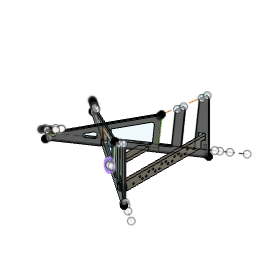
laptop-stand (Autodesk Fusion 360 design; units mm, degrees)
Autodesk Fusion 360 part; units mm, degrees
(part 1 of 2)
sketch "Side-Master" plane through (0, 0, 0) normal (0, 1, 0) x (1, 0, 0) in component "MainPanelRight"
  line L0 (8.1062, 0) -> (397.2, 0)
  line L1 (15.0761, -30.319) -> (18.2492, -20.8358)
  line L2 (13.8069, -34.1123) -> (25, -34.1123) construction
  line L3 (277.5681, -20) -> (310.5681, -20)
  line L4 (277.5681, -20) -> (284.9108, -103.9275)
  line L5 (277.5681, -20) -> (278, -20) construction
  line L6 (277.5681, -20) -> (277.5681, 0) construction
  line L7 (18.2492, -20.8358) -> (279.6598, -108.0704)
  line L8 (310.5681, -20) -> (428, -20) construction
  line L9 (332.9681, -20) -> (365.9681, -20)
  line L10 (365.9681, -20) -> (379.1493, -170.6626)
  line L11 (365.9681, -20) -> (495.2, -20) construction
  line L12 (381.4538, -174.4501) -> (395.0588, -183.0721) construction
  line L13 (401.2, -4) -> (401.2, -179.6934)
  line L14 (-0.6166, -29.9937) -> (35.0053, -29.9937) construction
  line L15 (13.8069, -34.1123) -> (37.7388, -34.1123) construction
  line L16 (13.8069, -34.1123) -> (-9.9012, -26.1797) construction
  line L17 (13.8069, -34.1123) -> (40, -34.1123) construction
  line L18 (0.3599, -26.0548) -> (4.1611, -3.3398)
  line L19 (-0.204, -29.4243) -> (25.3133, -29.4243) construction
  line L20 (3.0358, -30.5083) -> (10.0136, -32.8431)
  line L21 (0, 0) -> (138.5, 0) construction
  line L22 (138.5, 0) -> (138.5, -20.0011) construction
  line L23 (0, -20) -> (0, 0) construction
  line L24 (138.5, -20.0011) -> (138.4351, -60.9427) construction
  line L25 (147.5, -20.0011) -> (147.4778, -63.9603) construction
  line L26 (147.5, -20.0011) -> (147.5, 0) construction
  arc A0 (279.6598, -108.0704) -> (284.9108, -103.9275) centre (280.926, -104.2761) ccw
  arc A1 (379.1493, -170.6626) -> (381.4538, -174.4501) centre (384.1303, -170.2268) ccw
  arc A2 (395.0588, -183.0721) -> (401.2, -179.6934) centre (397.2, -179.6934) ccw
  arc A3 (401.2, -4) -> (397.2, 0) centre (397.2, -4) ccw
  arc A4 (0.3599, -26.0548) -> (3.0358, -30.5083) centre (4.305, -26.715) ccw
  arc A5 (8.1062, 0) -> (4.1611, -3.3398) centre (8.1062, -4) ccw
  arc A6 (10.0136, -32.8431) -> (15.0761, -30.319) centre (11.2828, -29.0498) ccw
  line L27 (285.442, -110) -> (379.1965, -169.4156) construction
  line L28 (310.5681, -20) -> (320.2067, -130.1699)
  line L29 (310.5681, -20) -> (415.8497, -20) construction
  line L30 (332.9681, -20) -> (343.3891, -139.1136)
  line L31 (332.9681, -20) -> (452.9694, -20) construction
  line L32 (322.0503, -133.1999) -> (337.2632, -142.8409)
  arc A7 (320.2067, -130.1699) -> (322.0503, -133.1999) centre (324.1914, -129.8213) ccw
  arc A8 (337.2632, -142.8409) -> (343.3891, -139.1136) centre (339.4044, -139.4622) ccw
  line L33 (381.4538, -174.4501) -> (395.0588, -183.0721)
  line L34 (278, -20) -> (0, -20) construction
  line L35 (310.5681, -20) -> (332.9681, -20) construction
  line L36 (277.5681, -20) -> (257.5681, -20) construction
  line L37 (257.5681, -20) -> (257.5681, -10) construction
  line L38 (257.5681, -10) -> (277.5681, -10) construction
  line L39 (277.5681, -10) -> (277.5681, -20) construction
  line L40 (395.2, -20) -> (390.2, -20) construction
  line L41 (390.2, -20) -> (390.2, -35) construction
  line L42 (390.2, -35) -> (395.2, -35) construction
  line L43 (395.2, -35) -> (395.2, -20) construction
  point P0 (401.2, 0)
  point P1 (285.442, -110)
  dimension "d1" = 401.2
  dimension "d5" = 30
  dimension "d8_1" = 15
  dimension "d9_1" = 71.5
  dimension "d10_1" = 14
  dimension "d11_1" = 33
  dimension "d12_1" = 85
  dimension "d14" = 20
  dimension "d15" = 90
  dimension "d24" = 33
  dimension "d25" = 85
  dimension "d26" = 150
  dimension "d41" = 161.5
  dimension "d42" = 25
  dimension "d44" = 80.5
  dimension "d66" = 138.5
  dimension "d67" = 20
  dimension "d68" = 9
  dimension "d129" = 4
  dimension "d130" = 5
  dimension "d131" = 4
  dimension "d134" = 4
  dimension "d137" = 4
  dimension "d138" = 4
  dimension "d139" = 4
  dimension "d140" = 85
  dimension "d141" = 85
  dimension "d142" = 4
  dimension "d143" = 4
  dimension "d146" = 22.4
  dimension "d38" = 20
  dimension "d39" = 10
  dimension "d53" = 5
  dimension "d54" = 15
  dimension "d156" = 6
  constraint horizontal L0
  constraint coincident L21.start L23.end
  constraint horizontal L2
  constraint horizontal L3
  constraint horizontal L5
  constraint coincident L0 L6.end
  constraint perpendicular L0 L6
  constraint horizontal L8
  constraint parallel L8 L9
  constraint horizontal L11
  constraint horizontal L14
  constraint horizontal L15
  constraint horizontal L17
  constraint horizontal L19
  constraint coincident L16 L19.start
  constraint horizontal L21
  constraint vertical L22
  constraint vertical L23
  constraint coincident L7 L24.end
  constraint coincident L7 L25.end
  constraint coincident L0 L26.end
  constraint perpendicular L0 L26
  constraint coincident P1 L7
  constraint coincident P1 L4
  constraint tangent L7 A0
  constraint tangent L4 A0
  constraint tangent L10 A1
  constraint tangent L12 A1
  constraint tangent L12 A2
  constraint tangent L13 A2
  constraint coincident P0 L13
  constraint coincident P0 L0
  constraint tangent L13 A3
  constraint tangent L0 A3
  constraint coincident L19.start L20
  constraint coincident L19.start L18
  constraint tangent L20 A4
  constraint tangent L18 A4
  constraint coincident L21.start L0
  constraint tangent L18 A5
  constraint tangent L0 A5
  constraint coincident L2.start L20
  constraint coincident L2.start L1
  constraint tangent L20 A6
  constraint tangent L1 A6
  constraint coincident P1 L27.start
  constraint horizontal L29
  constraint horizontal L31
  constraint tangent L28 A7
  constraint tangent L32 A7
  constraint tangent L32 A8
  constraint tangent L30 A8
  constraint perpendicular L23 L34
  constraint parallel L29 L35
  constraint collinear L27 L32
  constraint coincident L27.end A1
  constraint parallel L27 L33
  constraint horizontal L36
  constraint vertical L37
  constraint horizontal L38
  constraint vertical L39
  constraint horizontal L40
  constraint vertical L41
  constraint horizontal L42
  constraint vertical L43
  constraint coincident L31 L40.start
  constraint vertical L13
  measures "d1" distance of L21.start P0
  measures "d5" distance of L21.start L14.start
  measures "d8_1" distance of L14.start L2.start
  measures "d9_1" angle of L1 L2
  measures "d10_1" distance of L2.start L1.end
  measures "d11_1" distance of L3.start L3.end
  measures "d12_1" angle of L4 L5
  measures "d14" distance of L0 L3
  measures "d15" vertical distance of L3.start P1
  measures "d24" distance of L9.start L9.end
  measures "d25" angle of L10 L11
  measures "d26" distance of L9.end L27.end
  measures "d41" angle of L16 L17
  measures "d42" distance of L2.start L16.end
  measures "d44" angle of L18 L19
  measures "d66" distance of L21.start L21.end
  measures "d67" distance of L21.start L23.start
  measures "d68" distance of L22.end L25.start
  measures "d129" radius of A0
  measures "d130" radius of A1
  measures "d131" radius of A2
  measures "d134" radius of A3
  measures "d137" radius of A4
  measures "d138" radius of A5
  measures "d139" radius of A6
  measures "d140" angle of L28 L29
  measures "d141" angle of L30 L31
  measures "d142" radius of A7
  measures "d143" radius of A8
  measures "d146" distance of L3.end L9.start
  measures "d38" distance of L3.start L36.end
  measures "d39" distance of L3.start L38.end
  measures "d53" distance of L40.start L40.end
  measures "d54" distance of L40.start L42.end
  measures "d156" distance of L13 L43
extrude "Extrude24" add sketch "Side-Master" along normal mid plane 9 makes body 1 in component "MainPanelRight"
sketch "Sketch12" plane through (0, 0, 0) normal (0, 0, -1) x (1, 0, 0) in component "MainPanelRight"
  line L0 (8.1062, 4.5) -> (8.1062, -4.5)
  line L1 (8.1062, -4.5) -> (397.2, -4.5)
  line L2 (397.2, -4.5) -> (397.2, 4.5)
  line L3 (397.2, 4.5) -> (8.1062, 4.5)
  line L4 (397.2, 0) -> (401.2, 0) construction
  dimension "d149" = 4
  constraint midpoint L2 L4.start
  constraint perpendicular L2 L4
  measures "d149" distance of L4.start L4.end
sketch "Side-Master (2)" plane through (0, 0, 0) normal (0, 1, 0) x (1, 0, 0) in component "MainPanelLeft"
  line L0 (8.1062, 0) -> (397.2, 0)
  line L1 (15.0761, -30.319) -> (18.2492, -20.8358)
  line L2 (13.8069, -34.1123) -> (25, -34.1123) construction
  line L3 (277.5681, -20) -> (310.5681, -20)
  line L4 (277.5681, -20) -> (284.9108, -103.9275)
  line L5 (277.5681, -20) -> (278, -20) construction
  line L6 (277.5681, -20) -> (277.5681, 0) construction
  line L7 (18.2492, -20.8358) -> (279.6598, -108.0704)
  line L8 (310.5681, -20) -> (428, -20) construction
  line L9 (332.9681, -20) -> (365.9681, -20)
  line L10 (365.9681, -20) -> (379.1479, -170.6469)
  line L11 (365.9681, -20) -> (495.2, -20) construction
  line L12 (381.4524, -174.4344) -> (395.0587, -183.0577) construction
  line L13 (401.2, -4) -> (401.2, -179.6791)
  line L14 (-0.6166, -29.9937) -> (35.0053, -29.9937) construction
  line L15 (13.8069, -34.1123) -> (37.7388, -34.1123) construction
  line L16 (13.8069, -34.1123) -> (-9.9012, -26.1797) construction
  line L17 (13.8069, -34.1123) -> (40, -34.1123) construction
  line L18 (0.3599, -26.0548) -> (4.1611, -3.3398)
  line L19 (-0.204, -29.4243) -> (25.3133, -29.4243) construction
  line L20 (3.0358, -30.5083) -> (10.0136, -32.8431)
  line L21 (0, 0) -> (138.5, 0) construction
  line L22 (138.5, 0) -> (138.5, -20.0011) construction
  line L23 (0, -20) -> (0, 0) construction
  line L24 (138.5, -20.0011) -> (138.4351, -60.9427) construction
  line L25 (147.5, -20.0011) -> (147.4778, -63.9603) construction
  line L26 (147.5, -20.0011) -> (147.5, 0) construction
  arc A0 (279.6598, -108.0704) -> (284.9108, -103.9275) centre (280.926, -104.2761) ccw
  arc A1 (379.1479, -170.6469) -> (381.4524, -174.4344) centre (384.1289, -170.2111) ccw
  arc A2 (395.0587, -183.0577) -> (401.2, -179.6791) centre (397.2, -179.6791) ccw
  arc A3 (401.2, -4) -> (397.2, 0) centre (397.2, -4) ccw
  arc A4 (0.3599, -26.0548) -> (3.0358, -30.5083) centre (4.305, -26.715) ccw
  arc A5 (8.1062, 0) -> (4.1611, -3.3398) centre (8.1062, -4) ccw
  arc A6 (10.0136, -32.8431) -> (15.0761, -30.319) centre (11.2828, -29.0498) ccw
  line L27 (285.442, -110) -> (379.1926, -169.4159) construction
  line L28 (310.5681, -20) -> (320.2068, -130.1711)
  line L29 (310.5681, -20) -> (415.8497, -20) construction
  line L30 (332.9681, -20) -> (343.3893, -139.1153)
  line L31 (332.9681, -20) -> (452.9694, -20) construction
  line L32 (322.0503, -133.2011) -> (337.2633, -142.8425)
  arc A7 (320.2068, -130.1711) -> (322.0503, -133.2011) centre (324.1916, -129.8225) ccw
  arc A8 (337.2633, -142.8425) -> (343.3893, -139.1153) centre (339.4045, -139.4639) ccw
  line L33 (381.4524, -174.4344) -> (395.0587, -183.0577)
  line L34 (278, -20) -> (0, -20) construction
  line L35 (310.5681, -20) -> (332.9681, -20) construction
  line L36 (277.5681, -20) -> (257.5681, -20) construction
  line L37 (257.5681, -20) -> (257.5681, -10) construction
  line L38 (257.5681, -10) -> (277.5681, -10) construction
  line L39 (277.5681, -10) -> (277.5681, -20) construction
  line L40 (257.5681, -10) -> (247.5681, -10) construction
  line L41 (395.2, -20) -> (390.2, -20) construction
  line L42 (390.2, -20) -> (390.2, -35) construction
  line L43 (390.2, -35) -> (395.2, -35) construction
  line L44 (395.2, -35) -> (395.2, -20) construction
  line L45 (390.2, -35) -> (390.2, -45) construction
  point P0 (401.2, 0)
  point P1 (285.442, -110)
  dimension "d1_1" = 401.2
  dimension "d5_1" = 30
  dimension "d8_2" = 15
  dimension "d9_2" = 71.5
  dimension "d10_2" = 14
  dimension "d11_2" = 33
  dimension "d12_2" = 85
  dimension "d14_1" = 20
  dimension "d15_1" = 90
  dimension "d24_1" = 33
  dimension "d25_1" = 85
  dimension "d26_1" = 150
  dimension "d41_1" = 161.5
  dimension "d42_1" = 25
  dimension "d44_1" = 80.5
  dimension "d66_1" = 138.5
  dimension "d67_1" = 20
  dimension "d68_1" = 9
  dimension "d129_1" = 4
  dimension "d130_1" = 5
  dimension "d131_1" = 4
  dimension "d134_1" = 4
  dimension "d137_1" = 4
  dimension "d138_1" = 4
  dimension "d139_1" = 4
  dimension "d140_1" = 85
  dimension "d141_1" = 85
  dimension "d142_1" = 4
  dimension "d143_1" = 4
  dimension "d146_1" = 22.4
  dimension "d37" = 20
  dimension "d40" = 10
  dimension "d50" = 5
  dimension "d51" = 15
  dimension "d52" = 10
  dimension "d155" = 6
  constraint horizontal L0
  constraint coincident L21.start L23.end
  constraint horizontal L2
  constraint horizontal L3
  constraint horizontal L5
  constraint coincident L0 L6.end
  constraint perpendicular L0 L6
  constraint horizontal L8
  constraint parallel L8 L9
  constraint horizontal L11
  constraint horizontal L14
  constraint horizontal L15
  constraint horizontal L17
  constraint horizontal L19
  constraint coincident L16 L19.start
  constraint horizontal L21
  constraint vertical L22
  constraint vertical L23
  constraint coincident L7 L24.end
  constraint coincident L7 L25.end
  constraint coincident L0 L26.end
  constraint perpendicular L0 L26
  constraint coincident P1 L7
  constraint coincident P1 L4
  constraint tangent L7 A0
  constraint tangent L4 A0
  constraint tangent L10 A1
  constraint tangent L12 A1
  constraint tangent L12 A2
  constraint tangent L13 A2
  constraint coincident P0 L13
  constraint coincident P0 L0
  constraint tangent L13 A3
  constraint tangent L0 A3
  constraint coincident L19.start L20
  constraint coincident L19.start L18
  constraint tangent L20 A4
  constraint tangent L18 A4
  constraint coincident L21.start L0
  constraint tangent L18 A5
  constraint tangent L0 A5
  constraint coincident L2.start L20
  constraint coincident L2.start L1
  constraint tangent L20 A6
  constraint tangent L1 A6
  constraint coincident P1 L27.start
  constraint horizontal L29
  constraint horizontal L31
  constraint tangent L28 A7
  constraint tangent L32 A7
  constraint tangent L32 A8
  constraint tangent L30 A8
  constraint perpendicular L23 L34
  constraint parallel L29 L35
  constraint collinear L27 L32
  constraint coincident L27.end A1
  constraint parallel L27 L33
  constraint horizontal L36
  constraint vertical L37
  constraint horizontal L38
  constraint vertical L39
  constraint perpendicular L37 L40
  constraint horizontal L41
  constraint vertical L42
  constraint horizontal L43
  constraint vertical L44
  constraint coincident L29 L41.start
  constraint perpendicular L43 L45
  constraint vertical L13
  measures "d1_1" distance of L21.start P0
  measures "d5_1" distance of L21.start L14.start
  measures "d8_2" distance of L14.start L2.start
  measures "d9_2" angle of L1 L2
  measures "d10_2" distance of L2.start L1.end
  measures "d11_2" distance of L3.start L3.end
  measures "d12_2" angle of L4 L5
  measures "d14_1" distance of L0 L3
  measures "d15_1" vertical distance of L3.start P1
  measures "d24_1" distance of L9.start L9.end
  measures "d25_1" angle of L10 L11
  measures "d26_1" distance of L9.end L27.end
  measures "d41_1" angle of L16 L17
  measures "d42_1" distance of L2.start L16.end
  measures "d44_1" angle of L18 L19
  measures "d66_1" distance of L21.start L21.end
  measures "d67_1" distance of L21.start L23.start
  measures "d68_1" distance of L22.end L25.start
  measures "d129_1" radius of A0
  measures "d130_1" radius of A1
  measures "d131_1" radius of A2
  measures "d134_1" radius of A3
  measures "d137_1" radius of A4
  measures "d138_1" radius of A5
  measures "d139_1" radius of A6
  measures "d140_1" angle of L28 L29
  measures "d141_1" angle of L30 L31
  measures "d142_1" radius of A7
  measures "d143_1" radius of A8
  measures "d146_1" distance of L3.end L9.start
  measures "d37" distance of L3.start L36.end
  measures "d40" distance of L37.end L40.end
  measures "d50" distance of L41.start L41.end
  measures "d51" distance of L41.start L43.end
  measures "d52" distance of L42.end L45.end
  measures "d155" distance of L13 L44
extrude "Extrude24'" add sketch "Side-Master (2)" along normal mid plane 9 separate body makes body 2 in component "MainPanelLeft"
sketch "Sketch12 (2)" plane through (0, 0, 0) normal (0, 0, -1) x (1, 0, 0) in component "MainPanelLeft"
  line L0 (8.1062, 4.5) -> (8.1062, -4.5)
  line L1 (8.1062, -4.5) -> (397.2, -4.5)
  line L2 (397.2, -4.5) -> (397.2, 4.5)
  line L3 (397.2, 4.5) -> (8.1062, 4.5)
  line L4 (397.2, 0) -> (401.2, 0) construction
  dimension "d149_1" = 4
  constraint midpoint L2 L4.start
  constraint perpendicular L2 L4
  measures "d149_1" distance of L4.start L4.end
sketch "WidthAtBack" plane through (0, 0, 0) normal (0, 0, 1) x (1, 0, 0)
  line L0 (301.2084, 132.8518) -> (301.2084, -127.1482)
  dimension "d3" = 260
  constraint vertical L0
  measures "d3" distance of L0.start L0.end
sketch "CutOutOfPanels" plane through (-8.7916, 83.8613, 0) normal (0, 0, -1) x (0.826667, -0.562692, 0)
  line L0 (8.1062, 4.5) -> (8.1062, -4.5)
  line L1 (8.1062, -4.5) -> (397.2, -4.5)
  line L2 (397.2, -4.5) -> (397.2, 4.5)
  line L3 (397.2, 4.5) -> (8.1062, 4.5)
  line L4 (98.3262, 128.0447) -> (89.9533, 124.7439)
  line L5 (89.9533, 124.7439) -> (232.6556, -237.2368)
  line L6 (232.6556, -237.2368) -> (241.0285, -233.936)
  line L7 (241.0285, -233.936) -> (98.3262, 128.0447)
  line L8 (137.3566, 4.5) -> (137.3566, -4.5)
  line L9 (150.5788, -4.5) -> (142.2059, -7.8008)
  line L10 (137.3566, 4.5) -> (145.7295, 7.8008)
  line L11 (150.5788, -4.5) -> (150.5788, 4.5)
  line L12 (145.7295, 7.8008) -> (147.0308, 4.5)
  line L13 (147.0308, 4.5) -> (150.5788, 4.5)
  line L14 (142.2059, -7.8008) -> (140.9047, -4.5)
  line L15 (140.9047, -4.5) -> (137.3566, -4.5)
  constraint coincident L5 L8.start
  constraint coincident L3 L8.start
  constraint coincident L1 L8.end
  constraint perpendicular L1 L8
  constraint coincident L7 L9.start
  constraint coincident L1 L9.start
  constraint coincident L5 L9.end
  constraint perpendicular L5 L9
  constraint coincident L7 L10.end
  constraint perpendicular L7 L10
  constraint coincident L3 L11.end
  constraint perpendicular L3 L11
  constraint coincident L3 L12.end
  constraint coincident L7 L12.end
  constraint coincident L1 L14.end
  constraint coincident L5 L14.end
extrude "CutOutBottom" cut sketch "CutOutOfPanels" against normal blind 20 contours L3 L7 L10 L12 | L1 L3 L5 L7 | L1 L5 L8 L15 | L3 L7 L11 L13 | L1 L5 L9 L14 sketch seen with x (0.826667, -0.562692, 0) y (0.562692, 0.826667, 0) z (0, 0, 1) at (51.2464, 59.6633, 0) bodies 1 in component "MainPanelRight"
extrude "CutOutTop" cut sketch "CutOutOfPanels" against normal blind 100 from surface at -20 contours L3 L7 L10 L12 | L1 L3 L5 L7 | L1 L5 L8 L15 | L3 L7 L11 L13 | L1 L5 L9 L14 sketch seen with x (0.826667, 0.562692, 0) y (-0.562692, 0.826667, 0) z (0, 0, 1) at (54.4558, -64.3784, 0) bodies 2 in component "MainPanelLeft"
ref_plane "WorkPlane3" through (204.1313, -61.0702, 10) normal (0, 0, -1) x (-1, 0, 0)
sketch "MiddleStretchThing" plane through (204.1313, -61.0702, 10) normal (0, 0, -1) x (1, 0, 0)
  line L0 (-203.6897, -144.0902) -> (117.9612, 74.8498) construction
  line L1 (117.9612, -202.6937) -> (-203.6897, 16.2462) construction
  line L2 (0, 20) -> (0, -160) construction
  line L3 (-20, 20) -> (-20, -160) construction
  line L4 (112.897, 82.2898) -> (-208.7539, -136.6502) construction
  line L5 (-208.7539, 8.8062) -> (112.897, -210.1337) construction
  line L6 (-18.8746, -9.8233) -> (-14.9358, -15.61)
  line L7 (-14.9358, -15.61) -> (-20, -19.0571)
  line L8 (0, -5.4435) -> (-5.0642, -8.8906)
  line L9 (-5.0642, -8.8906) -> (-9.0031, -3.104)
  line L10 (-11.7818, -2.576) -> (-18.3467, -7.0446)
  line L11 (-20, -19.0571) -> (-20, -108.7869)
  line L12 (-18.7058, -117.7727) -> (-14.9358, -112.234)
  line L13 (-14.9358, -112.234) -> (-20, -108.7869)
  line L14 (0, -122.4004) -> (-5.0642, -118.9533)
  line L15 (-5.0642, -118.9533) -> (-8.8343, -124.492)
  line L16 (-12.0298, -125.0991) -> (-18.0987, -120.9682)
  line L17 (0, -122.4004) -> (0, -5.4435)
  arc A0 (-18.7058, -117.7727) -> (-18.0987, -120.9682) centre (-16.8045, -119.0669) ccw
  arc A1 (-12.0298, -125.0991) -> (-8.8343, -124.492) centre (-10.7356, -123.1978) ccw
  arc A2 (-18.3467, -7.0446) -> (-18.8746, -9.8233) centre (-17.2213, -8.6979) ccw
  arc A3 (-9.0031, -3.104) -> (-11.7818, -2.576) centre (-10.6564, -4.2294) ccw
  dimension "d46" = 2.3
  dimension "d47" = 2.3
  dimension "d48" = 2
  dimension "d49" = 2
  constraint vertical L2
  constraint vertical L3
  constraint coincident L0 L6.end
  constraint perpendicular L0 L6
  constraint coincident L3 L7.end
  constraint coincident L0 L7.end
  constraint coincident L2 L8.start
  constraint coincident L0 L8.start
  constraint coincident L0 L8.end
  constraint equal L7 L8
  constraint perpendicular L4 L9
  constraint coincident L1 L11.end
  constraint coincident L3 L11.end
  constraint coincident L1 L12.end
  constraint perpendicular L1 L12
  constraint coincident L1 L14.start
  constraint coincident L2 L14.start
  constraint coincident L1 L14.end
  constraint equal L13 L14
  constraint perpendicular L5 L15
  constraint tangent L12 A0
  constraint tangent L16 A0
  constraint tangent L16 A1
  constraint tangent L15 A1
  constraint tangent L10 A2
  constraint tangent L6 A2
  constraint tangent L10 A3
  constraint tangent L9 A3
  measures "d46" radius of A0
  measures "d47" radius of A1
  measures "d48" radius of A2
  measures "d49" radius of A3
extrude "Extrude2" add sketch "MiddleStretchThing" along normal mid plane 9 separate body makes body 3
ref_plane "WorkPlane5" through (313.7737, -135.7011, 35) normal (-1, 0, 0) x (0, -1, 0)
sketch "BackBarHelper" plane through (313.7737, -135.7011, 35) normal (-1, 0, 0) x (0, 1, 0)
  line L0 (277.104, -25) -> (13.2757, -24.9512)
  line L1 (0, 0) -> (-10.5021, 0)
  line L2 (-10.5021, 0) -> (-10.5021, -25)
  line L3 (-10.5021, -25) -> (4.498, -25)
  line L4 (277.104, -25) -> (288.2734, -25)
  line L5 (13.2757, -24.9512) -> (4.498, -25)
  line L6 (288.2734, -25) -> (288.2734, 0)
  line L7 (0, 0) -> (288.2734, 0)
  point P0 (277.1058, 0)
  dimension "d62" = 25
  dimension "d157" = 25
  dimension "d158" = 25
  constraint horizontal L1
  constraint vertical L2
  constraint horizontal L3
  constraint coincident L1.start L7.start
  constraint horizontal L4
  constraint perpendicular L4 L6
  measures "d62" distance of P0 L0.start
  measures "d157" distance of L4.end L6.end
  measures "d158" distance of L1.end L2.end
extrude "Extrude5" add sketch "BackBarHelper" along normal blind 9 separate body makes body 4
sketch "BackBar" plane through (313.7737, -135.7011, 35) normal (-1, 0, 0) x (0, 1, 0)
  line L0 (-5.4435, -14.9478) -> (-5.4435, -4.9478)
  line L1 (-5.4435, -4.9478) -> (-8.1435, -4.9478)
  line L2 (-10.4435, -7.2478) -> (-10.4435, -22.6478)
  line L3 (-8.1435, -24.9478) -> (-5.4435, -24.9478)
  line L4 (-5.4435, -14.9478) -> (11.5696, -14.9478)
  line L5 (11.5696, -14.9478) -> (11.5696, 4.9123)
  arc A0 (-10.4435, -22.6478) -> (-8.1435, -24.9478) centre (-8.1435, -22.6478) ccw
  arc A1 (-8.1435, -4.9478) -> (-10.4435, -7.2478) centre (-8.1435, -7.2478) ccw
  line L6 (-5.4435, -24.9478) -> (282.5494, -25.001)
  line L7 (282.5494, -25.001) -> (285.2494, -25.0015)
  line L8 (287.5498, -22.7019) -> (287.5527, -7.3019)
  line L9 (285.2531, -5.0015) -> (282.5531, -5.001)
  line L10 (282.5531, -5.001) -> (282.5512, -15.001)
  arc A2 (285.2494, -25.0015) -> (287.5498, -22.7019) centre (285.2498, -22.7015) ccw
  arc A3 (287.5527, -7.3019) -> (285.2531, -5.0015) centre (285.2527, -7.3015) ccw
  line L11 (282.5512, -15.001) -> (265.5362, -14.9979)
  line L12 (11.5696, 4.9123) -> (265.5362, 4.9123)
  line L13 (265.5362, 4.9123) -> (265.5362, -14.9979)
  line L14 (138.5529, -45.0877) -> (138.5529, 54.9123) construction
  line L15 (138.5529, -24.9744) -> (145.5529, -24.9744) construction
  line L16 (145.5529, -24.9744) -> (145.5529, -14.9744) construction
  line L17 (145.5529, -14.9744) -> (138.5529, -14.9744) construction
  line L18 (138.5529, -14.9744) -> (138.5529, -24.9744) construction
  line L19 (145.5529, -14.9744) -> (175.5529, -14.9744) construction
  line L20 (145.5529, -14.9744) -> (153.5529, -14.9744) construction
  line L21 (153.5529, -14.9744) -> (153.5529, -4.9744) construction
  line L22 (153.5529, -4.9744) -> (145.5529, -4.9744) construction
  line L23 (145.5529, -4.9744) -> (145.5529, -14.9744) construction
  line L24 (175.5529, -14.9744) -> (167.5529, -14.9744) construction
  line L25 (167.5529, -14.9744) -> (167.5529, -4.9744) construction
  line L26 (167.5529, -4.9744) -> (175.5529, -4.9744) construction
  line L27 (175.5529, -4.9744) -> (175.5529, -14.9744) construction
  line L28 (167.5529, -4.9744) -> (197.5529, -4.9744) construction
  line L29 (197.5529, -4.9744) -> (189.5529, -4.9744) construction
  line L30 (189.5529, -4.9744) -> (189.5529, -14.9744) construction
  line L31 (189.5529, -14.9744) -> (197.5529, -14.9744) construction
  line L32 (197.5529, -14.9744) -> (197.5529, -4.9744) construction
  line L33 (189.5529, -14.9744) -> (219.5529, -14.9744) construction
  line L34 (219.5529, -14.9744) -> (211.5529, -14.9744) construction
  line L35 (211.5529, -14.9744) -> (211.5529, -4.9744) construction
  line L36 (211.5529, -4.9744) -> (219.5529, -4.9744) construction
  line L37 (219.5529, -4.9744) -> (219.5529, -14.9744) construction
  line L38 (211.5529, -4.9744) -> (241.5529, -4.9744) construction
  circle A4 centre (145.5529, -14.9744) radius 3
  circle A5 centre (145.5529, -14.9744) radius 3
  circle A6 centre (153.5529, -4.9744) radius 3
  circle A7 centre (175.5529, -14.9744) radius 3
  circle A8 centre (175.5529, -14.9744) radius 3
  circle A9 centre (167.5529, -4.9744) radius 3
  circle A10 centre (197.5529, -4.9744) radius 3
  circle A11 centre (189.5529, -14.9744) radius 3
  circle A12 centre (219.5529, -14.9744) radius 3
  circle A13 centre (211.5529, -4.9744) radius 3
  circle A14 centre (241.5529, -4.9744) radius 3
  circle A15 centre (131.5529, -14.9744) radius 3
  circle A16 centre (123.5529, -4.9744) radius 3
  circle A17 centre (109.5529, -4.9744) radius 3
  circle A18 centre (101.5529, -14.9744) radius 3
  circle A19 centre (87.5529, -14.9744) radius 3
  circle A20 centre (79.5529, -4.9744) radius 3
  circle A21 centre (65.5529, -4.9744) radius 3
  circle A22 centre (57.5529, -14.9744) radius 3
  circle A23 centre (35.5529, -4.9744) radius 3
  point P0 (-5.4435, -24.9478)
  point P1 (-10.4435, -4.9478)
  point P2 (11.5696, -24.9509)
  point P3 (282.5494, -25.001)
  point P4 (276.4233, -24.9999)
  point P5 (287.5494, -25.0019)
  point P6 (287.5531, -5.0019)
  point P7 (271.6623, -24.999)
  point P8 (265.5362, -24.9979)
  dimension "d69" = 10
  dimension "d70" = 5
  dimension "d83" = 2.3
  dimension "d84" = 2.3
  dimension "d159" = 5
  dimension "d160" = 20
  dimension "d161" = 5
  dimension "d162" = 10
  dimension "d164" = 2.3
  dimension "d165" = 2.3
  dimension "d171" = 100
  dimension "d193" = 7
  dimension "d194" = 10
  dimension "d197" = 30
  dimension "d198" = 8
  dimension "d199" = 10
  dimension "d200" = 8
  dimension "d201" = 10
  dimension "d202" = 30
  dimension "d203" = 8
  dimension "d204" = 10
  dimension "d205" = 30
  dimension "d206" = 8
  dimension "d207" = 10
  dimension "d208" = 30
  dimension "d209" = 6
  dimension "d210" = 6
  dimension "d211" = 6
  dimension "d212" = 6
  dimension "d213" = 6
  dimension "d214" = 6
  dimension "d215" = 6
  dimension "d216" = 6
  dimension "d217" = 6
  dimension "d218" = 6
  dimension "d219" = 6
  constraint perpendicular L0 L1
  constraint perpendicular L1 L2
  constraint coincident P0 L3.end
  constraint perpendicular L0 L4
  constraint tangent L3 A0
  constraint tangent L2 A0
  constraint coincident P1 L1
  constraint coincident P1 L2
  constraint tangent L1 A1
  constraint tangent L2 A1
  constraint coincident P3 L6.end
  constraint parallel L6 L7
  constraint perpendicular L7 L8
  constraint perpendicular L8 L9
  constraint perpendicular L9 L10
  constraint coincident P5 L7
  constraint coincident P5 L8
  constraint tangent L7 A2
  constraint tangent L8 A2
  constraint coincident P6 L9
  constraint coincident P6 L8
  constraint tangent L9 A3
  constraint tangent L8 A3
  constraint perpendicular L10 L11
  constraint perpendicular L5 L12
  constraint vertical L13
  constraint vertical L14
  constraint midpoint L12 L14
  constraint horizontal L15
  constraint vertical L16
  constraint horizontal L17
  constraint vertical L18
  constraint midpoint L6 L15.start
  constraint perpendicular L16 L19
  constraint horizontal L20
  constraint vertical L21
  constraint horizontal L22
  constraint vertical L23
  constraint horizontal L24
  constraint vertical L25
  constraint horizontal L26
  constraint vertical L27
  constraint perpendicular L25 L28
  constraint horizontal L29
  constraint vertical L30
  constraint horizontal L31
  constraint vertical L32
  constraint perpendicular L30 L33
  constraint horizontal L34
  constraint vertical L35
  constraint horizontal L36
  constraint vertical L37
  constraint perpendicular L35 L38
  constraint coincident L16.end L17.start
  constraint coincident L25.end L26.start
  constraint coincident L28.end L29.start
  constraint coincident L30.end L31.start
  constraint coincident L33.end L34.start
  constraint coincident L35.end L36.start
  constraint coincident L38.end A14.centre
  constraint symmetric L14 A5 A15
  constraint symmetric L14 A6 A16
  constraint symmetric L14 A8 A18
  constraint symmetric L14 A9 A17
  constraint symmetric L14 A10 A20
  constraint symmetric L14 A11 A19
  constraint symmetric L14 A12 A22
  constraint symmetric L14 A13 A21
  constraint symmetric L14 A14 A23
  measures "d69" distance of L0.start L0.end
  measures "d70" distance of L0.end P1
  measures "d83" radius of A0
  measures "d84" radius of A1
  measures "d159" distance of P3 P5
  measures "d160" distance of P5 P6
  measures "d161" distance of P6 L9.end
  measures "d162" distance of L9.end L10.end
  measures "d164" radius of A2
  measures "d165" radius of A3
  measures "d171" distance of L14.start L14.end
  measures "d193" distance of L15.start L15.end
  measures "d194" distance of L15.start L17.end
  measures "d197" distance of L16.end L19.end
  measures "d198" distance of L16.end L20.end
  measures "d199" distance of L16.end L22.end
  measures "d200" distance of L19.end L24.end
  measures "d201" distance of L19.end L26.end
  measures "d202" distance of L25.end L28.end
  measures "d203" distance of L28.end L29.end
  measures "d204" distance of L28.end L31.end
  measures "d205" distance of L30.end L33.end
  measures "d206" distance of L33.end L34.end
  measures "d207" distance of L33.end L36.end
  measures "d208" distance of L35.end L38.end
  measures "d209" diameter of A4
  measures "d210" diameter of A5
  measures "d211" diameter of A6
  measures "d212" diameter of A7
  measures "d213" diameter of A8
  measures "d214" diameter of A9
  measures "d215" diameter of A10
  measures "d216" diameter of A11
  measures "d217" diameter of A12
  measures "d218" diameter of A13
  measures "d219" diameter of A14
extrude "Extrude6" add sketch "BackBar" along normal blind 9 separate body makes body 5
sketch "CutOutLeft" plane through (38.7573, 56.9394, 0) normal (0.562692, 0.826667, 0) x (-0.826667, 0.562692, 0)
  line L0 (-82.9008, 60.5828) -> (-82.9008, 20)
  line L1 (-82.9008, 20) -> (-96.123, 20)
  line L2 (-96.123, 20) -> (-96.123, 64.9951)
  line L3 (-96.123, 64.9951) -> (-225.2039, 108.0704)
  arc A0 (-225.2039, 108.0704) -> (-230.4549, 103.9275) centre (-226.4701, 104.2761) ccw
  line L4 (-230.4549, 103.9275) -> (-223.1122, 20)
  line L5 (-223.1122, 20) -> (-256.1122, 20)
  line L6 (-256.1122, 20) -> (-265.7509, 130.1711)
  arc A1 (-265.7509, 130.1711) -> (-267.5945, 133.2011) centre (-269.7357, 129.8225) ccw
  line L7 (-267.5945, 133.2011) -> (-282.8074, 142.8425)
  arc A2 (-282.8074, 142.8425) -> (-288.9334, 139.1153) centre (-284.9487, 139.4639) ccw
  line L8 (-288.9334, 139.1153) -> (-278.5122, 20)
  line L9 (-278.5122, 20) -> (-311.5122, 20)
  line L10 (-311.5122, 20) -> (-324.6921, 170.6469)
  arc A3 (-324.6921, 170.6469) -> (-326.9965, 174.4344) centre (-329.6731, 170.2111) ccw
  line L11 (-326.9965, 174.4344) -> (-340.6029, 183.0577)
  arc A4 (-340.6029, 183.0577) -> (-346.7442, 179.6791) centre (-342.7442, 179.6791) ccw
  line L12 (-346.7442, 179.6791) -> (-346.7442, 4)
  arc A5 (-346.7442, 4) -> (-342.7442, 0) centre (-342.7442, 4) ccw
  line L13 (-342.7442, 0) -> (46.3496, 0)
  arc A6 (46.3496, 0) -> (50.2947, 3.3398) centre (46.3496, 4) ccw
  line L14 (50.2947, 3.3398) -> (54.0959, 26.0548)
  arc A7 (54.0959, 26.0548) -> (51.42, 30.5083) centre (50.1508, 26.715) ccw
  line L15 (51.42, 30.5083) -> (44.4422, 32.8431)
  arc A8 (44.4422, 32.8431) -> (39.3797, 30.319) centre (43.173, 29.0498) ccw
  line L16 (39.3797, 30.319) -> (36.2067, 20.8358)
  line L17 (-321.794, 55) -> (-321.794, 70.9478)
  line L18 (-321.794, 70.9478) -> (-338.8072, 70.9478)
  line L19 (-338.8072, 70.9478) -> (-338.8072, 59.9478)
  line L20 (-321.794, 65) -> (-321.794, 49.9478)
  line L21 (-321.794, 49.9478) -> (-338.8072, 49.9478)
  line L22 (-338.8072, 49.9478) -> (-338.8072, 59.9478)
  line L23 (36.2067, 20.8358) -> (-82.9008, 60.5828)
  point P0 (-338.8072, 59.9478)
  point P1 (-321.794, 59.9509)
  dimension "d73" = 11
  dimension "d74" = 10
  constraint vertical L17
  constraint horizontal L18
  constraint vertical L19
  constraint coincident P0 L19.end
  constraint vertical L20
  constraint horizontal L21
  constraint vertical L22
  constraint coincident P1 L20
  constraint coincident P1 L17
  measures "d73" distance of P0 L18.end
  measures "d74" distance of P0 L21.end
extrude "Extrude27" cut sketch "CutOutLeft" against normal blind 9 contours L17 L18 L19 L20 L21 L22 sketch seen with x (0.826667, 0.562692, 0) y (-0.562692, 0.826667, 0) z (0, 0, 1) at (54.4558, -64.3784, 0) bodies 2 in component "MainPanelLeft"
sketch "CutOutRight" plane through (36.1042, -53.0417, 0) normal (0.562692, -0.826667, 0) x (0.826667, 0.562692, 0)
  line L0 (86.1102, 0) -> (86.1102, 20)
  line L1 (86.1102, 20) -> (99.3324, 20)
  line L2 (99.3324, 20) -> (99.3324, 0)
  line L3 (99.3324, 0) -> (345.9536, 0)
  arc A0 (345.9536, 0) -> (349.9536, 4) centre (345.9536, 4) ccw
  line L4 (349.9536, 4) -> (349.9536, 179.6934)
  arc A1 (349.9536, 179.6934) -> (343.8124, 183.0721) centre (345.9536, 179.6934) ccw
  line L5 (343.8124, 183.0721) -> (330.2074, 174.4501)
  arc A2 (330.2074, 174.4501) -> (327.9029, 170.6626) centre (332.8838, 170.2268) ccw
  line L6 (327.9029, 170.6626) -> (314.7216, 20)
  line L7 (314.7216, 20) -> (281.7216, 20)
  line L8 (281.7216, 20) -> (292.1427, 139.1136)
  arc A3 (292.1427, 139.1136) -> (286.0167, 142.8409) centre (288.1579, 139.4622) ccw
  line L9 (286.0167, 142.8409) -> (270.8038, 133.1999)
  arc A4 (270.8038, 133.1999) -> (268.9602, 130.1699) centre (272.945, 129.8213) ccw
  line L10 (268.9602, 130.1699) -> (259.3216, 20)
  line L11 (259.3216, 20) -> (226.3216, 20)
  line L12 (226.3216, 20) -> (233.6643, 103.9275)
  arc A5 (233.6643, 103.9275) -> (228.4133, 108.0704) centre (229.6795, 104.2761) ccw
  line L13 (228.4133, 108.0704) -> (-32.9973, 20.8358)
  line L14 (-32.9973, 20.8358) -> (-36.1703, 30.319)
  arc A6 (-36.1703, 30.319) -> (-41.2328, 32.8431) centre (-39.9636, 29.0498) ccw
  line L15 (-41.2328, 32.8431) -> (-48.2106, 30.5083)
  arc A7 (-48.2106, 30.5083) -> (-50.8865, 26.0548) centre (-46.9414, 26.715) ccw
  line L16 (-50.8865, 26.0548) -> (-47.0854, 3.3398)
  arc A8 (-47.0854, 3.3398) -> (-43.1402, 0) centre (-43.1402, 4) ccw
  line L17 (342.0166, 50.001) -> (325.0034, 50.001)
  line L18 (325.0034, 50.001) -> (325.0034, 71.001)
  line L19 (325.0034, 71.001) -> (342.0166, 71.001)
  line L20 (342.0166, 71.001) -> (342.0166, 50.001)
  line L21 (-43.1402, 0) -> (86.1102, 0)
  point P0 (342.0166, 50.001)
  point P1 (325.0034, 49.9979)
  dimension "d166" = 21
  constraint horizontal L17
  constraint vertical L18
  constraint horizontal L19
  constraint vertical L20
  constraint coincident P0 L17.start
  measures "d166" distance of P0 L19.end
extrude "Extrude28" cut sketch "CutOutRight" against normal blind 9 contours L17 L18 L19 L20 sketch seen with x (0.826667, -0.562692, 0) y (0.562692, 0.826667, 0) z (0, 0, 1) at (51.2464, 59.6633, 0) bodies 1 in component "MainPanelRight"
sketch "Sketch13" plane through (0, 4.5, 0) normal (0, 1, 0) x (-1, 0, 0) in component "MainPanelRight"
  line L0 (-137.3566, 20) -> (-137.3566, 0)
  line L1 (-137.3566, 0) -> (-8.1062, 0)
  arc A0 (-8.1062, 0) -> (-4.1611, 3.3398) centre (-8.1062, 4) ccw
  line L2 (-4.1611, 3.3398) -> (-0.3599, 26.0548)
  arc A1 (-0.3599, 26.0548) -> (-3.0358, 30.5083) centre (-4.305, 26.715) ccw
  line L3 (-3.0358, 30.5083) -> (-10.0136, 32.8431)
  arc A2 (-10.0136, 32.8431) -> (-15.0761, 30.319) centre (-11.2828, 29.0498) ccw
  line L4 (-15.0761, 30.319) -> (-18.2492, 20.8358)
  line L5 (-18.2492, 20.8358) -> (-279.6598, 108.0704)
  arc A3 (-279.6598, 108.0704) -> (-284.9108, 103.9275) centre (-280.926, 104.2761) ccw
  line L6 (-284.9108, 103.9275) -> (-277.5681, 20)
  line L7 (-277.5681, 20) -> (-310.5681, 20)
  line L8 (-310.5681, 20) -> (-320.2067, 130.1699)
  arc A4 (-320.2067, 130.1699) -> (-322.0503, 133.1999) centre (-324.1914, 129.8213) ccw
  line L9 (-322.0503, 133.1999) -> (-337.2632, 142.8409)
  arc A5 (-337.2632, 142.8409) -> (-343.3891, 139.1136) centre (-339.4044, 139.4622) ccw
  line L10 (-343.3891, 139.1136) -> (-332.9681, 20)
  line L11 (-332.9681, 20) -> (-365.9681, 20)
  line L12 (-365.9681, 20) -> (-379.1493, 170.6626)
  arc A6 (-379.1493, 170.6626) -> (-381.4538, 174.4501) centre (-384.1303, 170.2268) ccw
  line L13 (-381.4538, 174.4501) -> (-395.0588, 183.0721)
  arc A7 (-395.0588, 183.0721) -> (-401.2, 179.6934) centre (-397.2, 179.6934) ccw
  line L14 (-401.2, 179.6934) -> (-401.2, 4)
  arc A8 (-401.2, 4) -> (-397.2, 0) centre (-397.2, 4) ccw
  line L15 (-397.2, 0) -> (-150.5788, 0)
  line L16 (-150.5788, 0) -> (-150.5788, 20)
  line L17 (-150.5788, 20) -> (-137.3566, 20)
  line L18 (-150.5788, 0) -> (-160.5788, 0) construction
  line L19 (-160.5788, 0) -> (-160.5788, 20) construction
  line L20 (-160.5788, 20) -> (-150.5788, 20) construction
  line L21 (-150.5788, 20) -> (-150.5788, 0) construction
  line L22 (-277.5681, 20) -> (-284.9108, 103.9275) construction
  line L23 (-272.1074, 123.9538) -> (-263.5113, 25.699) construction
  line L24 (-294.9257, 97.8787) -> (13.9908, -5.209) construction
  line L25 (-18.2492, 20.8358) -> (-279.6598, 108.0704) construction
  line L26 (-277.5681, 20) -> (25, 20) construction
  line L27 (-160.5788, 20) -> (-160.5788, 48.7231) construction
  line L28 (-268.2744, 80.1422) -> (-263.5113, 25.699)
  line L29 (-257.5478, 20.222) -> (-166.5925, 20.0138)
  line L30 (-160.5788, 26.0138) -> (-160.5788, 48.7231)
  line L31 (-164.6795, 54.4146) -> (-260.398, 86.3566)
  arc A9 (-260.398, 86.3566) -> (-268.2744, 80.1422) centre (-262.2973, 80.6651) ccw
  arc A10 (-166.5925, 20.0138) -> (-160.5788, 26.0138) centre (-166.5788, 26.0138) ccw
  line L32 (-127.3566, -10) -> (-127.3566, 76) construction
  line L33 (-119.4574, 39.3236) -> (-96.5865, 31.6915)
  line L34 (-98.4858, 20) -> (-121.3566, 20)
  line L35 (-127.3566, 26) -> (-127.3566, 33.6322)
  arc A11 (-119.4574, 39.3236) -> (-127.3566, 33.6322) centre (-121.3566, 33.6322) ccw
  arc A12 (-98.4858, 20) -> (-96.5865, 31.6915) centre (-98.4858, 26) ccw
  arc A13 (-127.3566, 26) -> (-121.3566, 20) centre (-121.3566, 26) ccw
  line L36 (-376.2499, 71.001) -> (-376.2499, 50.001)
  line L37 (-376.2499, 50.001) -> (-393.263, 50.001)
  line L38 (-393.263, 50.001) -> (-393.263, 71.001)
  line L39 (-393.263, 71.001) -> (-376.2499, 71.001)
  arc A14 (-160.5788, 48.7231) -> (-164.6795, 54.4146) centre (-166.5788, 48.7231) ccw
  arc A15 (-263.5113, 25.699) -> (-257.5478, 20.222) centre (-257.5341, 26.222) ccw
  dimension "d91" = 10
  dimension "d92" = 20
  dimension "d98" = 14.5
  dimension "d99" = 14.5
  dimension "d100" = 6
  dimension "d101" = 6
  dimension "d113" = 10
  dimension "d114" = 6
  dimension "d115" = 6
  dimension "d116" = 6
  dimension "d223" = 6
  dimension "d224" = 6
  constraint horizontal L18
  constraint vertical L19
  constraint horizontal L20
  constraint vertical L21
  constraint coincident L15.end L16.start
  constraint parallel L22 L23
  constraint parallel L24 L25
  constraint coincident L6.end L7.start
  constraint horizontal L26
  constraint perpendicular L26 L27
  constraint tangent L28 A9
  constraint tangent L31 A9
  constraint coincident L19.end L29
  constraint coincident L19.end L30
  constraint tangent L29 A10
  constraint tangent L30 A10
  constraint vertical L32
  constraint tangent L33 A11
  constraint tangent L35 A11
  constraint tangent L33 A12
  constraint tangent L34 A12
  constraint tangent L35 A13
  constraint tangent L34 A13
  constraint collinear L24 L31
  constraint collinear L23 L28
  constraint collinear L24 L33
  constraint collinear L26 L34
  constraint collinear L32 L35
  constraint tangent L31 A14
  constraint tangent L27 A14
  constraint tangent L29 A15
  constraint tangent L23 A15
  measures "d91" distance of L15.end L18.end
  measures "d92" distance of L15.end L16.end
  measures "d98" distance of L22 L23
  measures "d99" distance of L24 L25
  measures "d100" radius of A9
  measures "d101" radius of A10
  measures "d113" distance of L0 L32
  measures "d114" radius of A11
  measures "d115" radius of A12
  measures "d116" radius of A13
  measures "d223" radius of A14
  measures "d224" radius of A15
extrude "Extrude29" cut sketch "Sketch13" against normal blind 9 contours L28 L29 L30 L31 A9 A10 A14 A15 | L33 L34 L35 A11 A12 A13 bodies 1 in component "MainPanelRight"
sketch "Sketch20" plane through (33.6931, 49.4994, 0) normal (-0.562692, -0.826667, 0) x (0.826667, -0.562692, 0)
  line L0 (321.794, 70.9478) -> (338.8072, 70.9478)
  line L1 (338.8072, 70.9478) -> (338.8072, 49.9478)
  line L2 (338.8072, 49.9478) -> (321.794, 49.9478)
  line L3 (82.9008, 20) -> (82.9008, 60.5828)
  line L4 (82.9008, 60.5828) -> (-36.2067, 20.8358)
  line L5 (-36.2067, 20.8358) -> (-39.3797, 30.319)
  arc A0 (-39.3797, 30.319) -> (-44.4422, 32.8431) centre (-43.173, 29.0498) ccw
  line L6 (-44.4422, 32.8431) -> (-51.42, 30.5083)
  arc A1 (-51.42, 30.5083) -> (-54.0959, 26.0548) centre (-50.1508, 26.715) ccw
  line L7 (-54.0959, 26.0548) -> (-50.2947, 3.3398)
  arc A2 (-50.2947, 3.3398) -> (-46.3496, 0) centre (-46.3496, 4) ccw
  line L8 (-46.3496, 0) -> (342.7442, 0)
  arc A3 (342.7442, 0) -> (346.7442, 4) centre (342.7442, 4) ccw
  line L9 (346.7442, 4) -> (346.7442, 179.6791)
  arc A4 (346.7442, 179.6791) -> (340.6029, 183.0577) centre (342.7442, 179.6791) ccw
  line L10 (340.6029, 183.0577) -> (326.9965, 174.4344)
  arc A5 (326.9965, 174.4344) -> (324.6921, 170.6469) centre (329.6731, 170.2111) ccw
  line L11 (324.6921, 170.6469) -> (311.5122, 20)
  line L12 (311.5122, 20) -> (278.5122, 20)
  line L13 (278.5122, 20) -> (288.9334, 139.1153)
  arc A6 (288.9334, 139.1153) -> (282.8074, 142.8425) centre (284.9487, 139.4639) ccw
  line L14 (282.8074, 142.8425) -> (267.5945, 133.2011)
  arc A7 (267.5945, 133.2011) -> (265.7509, 130.1711) centre (269.7357, 129.8225) ccw
  line L15 (265.7509, 130.1711) -> (256.1122, 20)
  line L16 (256.1122, 20) -> (223.1122, 20)
  line L17 (223.1122, 20) -> (230.4549, 103.9275)
  arc A8 (230.4549, 103.9275) -> (225.2039, 108.0704) centre (226.4701, 104.2761) ccw
  line L18 (225.2039, 108.0704) -> (96.123, 64.9951)
  line L19 (96.123, 64.9951) -> (96.123, 20)
  line L20 (96.123, 20) -> (82.9008, 20)
  line L21 (42.1307, 31.6915) -> (350.4016, 134.5638) construction
  line L22 (-36.2067, 20.8358) -> (225.2039, 108.0704) construction
  line L23 (213.8186, 80.1422) -> (204.144, -30.4389) construction
  line L24 (223.1122, 20) -> (230.4549, 103.9275) construction
  line L25 (203.0588, 20) -> (-70, 20) construction
  line L26 (214.6155, 89.2509) -> (209.036, 25.4771)
  line L27 (106.123, 100.05) -> (106.123, 26) construction
  line L28 (110.2237, 54.4146) -> (205.9421, 86.3566)
  line L29 (208.5568, 20) -> (112.123, 20)
  line L30 (106.123, 20) -> (106.123, 48.7231)
  arc A9 (213.8186, 80.1422) -> (205.9421, 86.3566) centre (207.8414, 80.6651) ccw
  arc A10 (203.0588, 20) -> (209.036, 25.4771) centre (203.0588, 26) ccw
  arc A11 (106.123, 26) -> (112.123, 20) centre (112.123, 26) ccw
  arc A12 (110.2237, 54.4146) -> (106.123, 48.7231) centre (112.123, 48.7231) ccw
  line L31 (72.9008, 33.6322) -> (72.9008, -24.4898) construction
  line L32 (321.794, 49.9478) -> (321.794, 70.9478)
  line L33 (72.9008, 41.9597) -> (72.9008, 26)
  line L34 (66.9008, 20) -> (44.03, 20)
  line L35 (7.0956, 20) -> (65.0015, 39.3236)
  arc A13 (72.9008, 33.6322) -> (65.0015, 39.3236) centre (66.9008, 33.6322) ccw
  arc A14 (42.1307, 31.6915) -> (44.03, 20) centre (44.03, 26) ccw
  arc A15 (66.9008, 20) -> (72.9008, 26) centre (66.9008, 26) ccw
  dimension "d104" = 14.5
  dimension "d105" = 14.5
  dimension "d106" = 10
  dimension "d107" = 6
  dimension "d108" = 6
  dimension "d109" = 6
  dimension "d117" = 10
  dimension "d220" = 6
  dimension "d221" = 6
  dimension "d222" = 6
  dimension "d225" = 20
  constraint parallel L21 L22
  constraint parallel L23 L24
  constraint perpendicular L9 L25
  constraint coincident L21 L26.start
  constraint coincident L23 L26.start
  constraint coincident L25 L29.start
  constraint coincident L23 L29.start
  constraint parallel L19 L27
  constraint coincident L25 L30.start
  constraint coincident L27 L30.start
  constraint coincident L26.start L28
  constraint tangent L28 A9
  constraint tangent L23 A9
  constraint coincident L29.start L26
  constraint tangent L26 A10
  constraint tangent L25 A10
  constraint equal A9 A10
  constraint coincident L30.start L29
  constraint tangent L27 A11
  constraint tangent L29 A11
  constraint tangent L28 A12
  constraint tangent L30 A12
  constraint parallel L3 L31
  constraint collinear L21 L28
  constraint parallel L27 L30
  constraint coincident L21 L33.start
  constraint coincident L31 L33.start
  constraint coincident L21 L35.start
  constraint coincident L25 L35.start
  constraint coincident L33.start L35
  constraint tangent L31 A13
  constraint tangent L35 A13
  constraint coincident L35.start L34
  constraint tangent L21 A14
  constraint tangent L34 A14
  constraint tangent L34 A15
  constraint tangent L33 A15
  measures "d104" distance of L21 L22
  measures "d105" distance of L23 L24
  measures "d106" distance of L19 L27
  measures "d107" radius of A9
  measures "d108" radius of A11
  measures "d109" radius of A12
  measures "d117" distance of L3 L31
  measures "d220" radius of A13
  measures "d221" radius of A14
  measures "d222" radius of A15
  measures "d225" distance of L8 L25
extrude "Extrude28'" cut sketch "Sketch20" against normal blind 9 contours L26 L28 L29 L30 A9 A10 A11 A12 | L33 L34 L35 A13 A14 A15 sketch seen with x (0.826667, 0.562692, 0) y (-0.562692, 0.826667, 0) z (0, 0, 1) at (54.4558, -64.3784, 0) bodies 2 in component "MainPanelLeft"